Autodesk Fusion 360 part; units mm, degrees
note: some values were not read from the file. Set by a fixed rule: which sketch regions a step uses.
(part 11 of 59)
  spline S58 degree 5 poles (-18.7406, 34.6904) (-18.7407, 34.6905) (-18.7408, 34.6907) (-18.741, 34.6909) (-18.7414, 34.6913) (-18.7419, 34.6919) (-18.7424, 34.6925) (-18.7431, 34.6933) (-18.7438, 34.6941) (-18.7446, 34.695) (-18.7455, 34.696) (-18.7464, 34.697) (-18.7474, 34.6982) (-18.7485, 34.6994) (-18.7497, 34.7007) (-18.7509, 34.702) (-18.7522, 34.7035) (-18.7536, 34.705) (-18.755, 34.7066) (-18.7565, 34.7082) (-18.7581, 34.7099) (-18.7597, 34.7117) (-18.7615, 34.7136) (-18.7632, 34.7155) (-18.7651, 34.7175) (-18.767, 34.7195) (-18.769, 34.7216) (-18.771, 34.7238) (-18.7732, 34.726) (-18.7753, 34.7283) (-18.7776, 34.7307) (-18.7799, 34.7331) (-18.7823, 34.7355) (-18.7847, 34.738) (-18.7872, 34.7406) (-18.7897, 34.7433) (-18.7924, 34.7459) (-18.7951, 34.7487) (-18.7978, 34.7515) (-18.8006, 34.7543) (-18.8035, 34.7572) (-18.8064, 34.7602) (-18.8094, 34.7632) (-18.8124, 34.7662) (-18.8156, 34.7693) (-18.8187, 34.7725) (-18.822, 34.7757) (-18.8252, 34.7789) (-18.8286, 34.7822) (-18.832, 34.7855) (-18.8355, 34.7889) (-18.839, 34.7923) (-18.8426, 34.7958) (-18.8462, 34.7993) (-18.8499, 34.8029) (-18.8536, 34.8065) (-18.8574, 34.8101) (-18.8613, 34.8138) (-18.8652, 34.8175) (-18.8692, 34.8212) (-18.8732, 34.825) (-18.8773, 34.8289) (-18.8814, 34.8328) (-18.8856, 34.8367) (-18.8899, 34.8406) (-18.8942, 34.8446) (-18.8986, 34.8486) (-18.903, 34.8527) (-18.9074, 34.8568) (-18.9119, 34.8609) (-18.9165, 34.8651) (-18.9211, 34.8693) (-18.9258, 34.8736) (-18.9306, 34.8778) (-18.9353, 34.8821) (-18.9402, 34.8865) (-18.9451, 34.8909) (-18.95, 34.8953) (-18.955, 34.8997) (-18.96, 34.9042) (-18.9651, 34.9087) (-18.9703, 34.9132) (-18.9755, 34.9177) (-18.9807, 34.9223) (-18.986, 34.927) (-18.9914, 34.9316) (-18.9968, 34.9363) (-19.0022, 34.941) (-19.0077, 34.9457) (-19.0133, 34.9505) (-19.0189, 34.9553) (-19.0246, 34.9601) (-19.0303, 34.9649) (-19.036, 34.9698) (-19.0418, 34.9747) (-19.0477, 34.9796) (-19.0536, 34.9846) (-19.0595, 34.9895) (-19.0655, 34.9945) (-19.0715, 34.9996) (-19.0776, 35.0046) (-19.0838, 35.0097) (-19.09, 35.0148) (-19.0962, 35.0199) (-19.1025, 35.025) (-19.1088, 35.0302) (-19.1152, 35.0354) (-19.1216, 35.0406) (-19.1281, 35.0458) (-19.1346, 35.0511) (-19.1412, 35.0564) (-19.1478, 35.0617) (-19.1544, 35.067) (-19.1611, 35.0723) (-19.1679, 35.0777) (-19.1747, 35.083) (-19.1815, 35.0884) (-19.1884, 35.0939) (-19.1954, 35.0993) (-19.2024, 35.1048) (-19.2094, 35.1102) (-19.2165, 35.1157) (-19.2236, 35.1212) (-19.2307, 35.1268) (-19.2379, 35.1323) (-19.2452, 35.1379) (-19.2525, 35.1435) (-19.2598, 35.1491) (-19.2672, 35.1547) (-19.2747, 35.1603) (-19.2821, 35.166) (-19.2897, 35.1716) (-19.2972, 35.1773) (-19.3048, 35.183) (-19.3125, 35.1887) (-19.3202, 35.1945) (-19.3279, 35.2002) (-19.3357, 35.206) (-19.3436, 35.2118) (-19.3514, 35.2175) (-19.3593, 35.2233) (-19.3673, 35.2292) (-19.3753, 35.235) (-19.3834, 35.2408) (-19.3914, 35.2467) (-19.3996, 35.2526) (-19.4078, 35.2585) (-19.416, 35.2644) (-19.4242, 35.2703) (-19.4325, 35.2762) (-19.4409, 35.2822) (-19.4493, 35.2881) (-19.4577, 35.2941) (-19.4662, 35.3) (-19.4747, 35.306) (-19.4832, 35.312) (-19.4918, 35.318) (-19.5005, 35.3241) (-19.5091, 35.3301) (-19.5179, 35.3361) (-19.5266, 35.3422) (-19.5354, 35.3483) (-19.5443, 35.3543) (-19.5532, 35.3604) (-19.5621, 35.3665) (-19.5711, 35.3726) (-19.5801, 35.3787) (-19.5891, 35.3849) (-19.5982, 35.391) (-19.6073, 35.3971) (-19.6165, 35.4033) (-19.6257, 35.4095) (-19.635, 35.4156) (-19.6443, 35.4218) (-19.6536, 35.428) (-19.663, 35.4342) (-19.6724, 35.4404) (-19.6818, 35.4466) (-19.6913, 35.4528) (-19.7009, 35.4591) (-19.7104, 35.4653) (-19.72, 35.4715) (-19.7297, 35.4778) (-19.7394, 35.484) (-19.7491, 35.4903) (-19.7589, 35.4966) (-19.7687, 35.5029) (-19.7785, 35.5091) (-19.7884, 35.5154) (-19.7984, 35.5217) (-19.8083, 35.528) (-19.8183, 35.5343) (-19.8284, 35.5406) (-19.8384, 35.547) (-19.8486, 35.5533) (-19.8587, 35.5596) (-19.8689, 35.566) (-19.8791, 35.5723) (-19.8894, 35.5786) (-19.8997, 35.585) (-19.9101, 35.5914) (-19.9205, 35.5977) (-19.9309, 35.6041) (-19.9413, 35.6104) (-19.9518, 35.6168) (-19.9624, 35.6232) (-19.973, 35.6296) (-19.9836, 35.636) (-19.9942, 35.6423) (-20.0049, 35.6487) (-20.0156, 35.6551) (-20.0264, 35.6615) (-20.0372, 35.6679) (-20.048, 35.6743) (-20.0589, 35.6807) (-20.0698, 35.6872) (-20.0808, 35.6936) (-20.0917, 35.7) (-20.1028, 35.7064) (-20.1138, 35.7128) (-20.1249, 35.7193) (-20.136, 35.7257) (-20.1472, 35.7321) (-20.1584, 35.7385) (-20.1697, 35.745) (-20.1809, 35.7514) (-20.1922, 35.7578) (-20.2036, 35.7643) (-20.215, 35.7707) (-20.2264, 35.7771) (-20.2379, 35.7836) (-20.2493, 35.79) (-20.2609, 35.7965) (-20.2724, 35.8029) (-20.284, 35.8094) (-20.2957, 35.8158) (-20.3073, 35.8222) (-20.319, 35.8287) (-20.3308, 35.8351) (-20.3426, 35.8416) (-20.3544, 35.848) (-20.3639, 35.8532) (-20.371, 35.8571) (-20.3757, 35.8596) (-20.3781, 35.8609) knots 0 0 0 0 0 0 0.00416667 0.00833333 0.0125 0.01666667 0.02083333 0.025 0.02916667 0.03333333 0.0375 0.04166667 0.04583333 0.05 0.05416667 0.05833333 0.0625 0.06666667 0.07083333 0.075 0.07916667 0.08333333 0.0875 0.09166667 0.09583333 0.1 0.10416667 0.10833333 0.1125 0.11666667 0.12083333 0.125 0.12916667 0.13333333 0.1375 0.14166667 0.14583333 0.15 0.15416667 0.15833333 0.1625 0.16666667 0.17083333 0.175 0.17916667 0.18333333 0.1875 0.19166667 0.19583333 0.2 0.20416667 0.20833333 0.2125 0.21666667 0.22083333 0.225 0.22916667 0.23333333 0.2375 0.24166667 0.24583333 0.25 0.25416667 0.25833333 0.2625 0.26666667 0.27083333 0.275 0.27916667 0.28333333 0.2875 0.29166667 0.29583333 0.3 0.30416667 0.30833333 0.3125 0.31666667 0.32083333 0.325 0.32916667 0.33333333 0.3375 0.34166667 0.34583333 0.35 0.35416667 0.35833333 0.3625 0.36666667 0.37083333 0.375 0.37916667 0.38333333 0.3875 0.39166667 0.39583333 0.4 0.40416667 0.40833333 0.4125 0.41666667 0.42083333 0.425 0.42916667 0.43333333 0.4375 0.44166667 0.44583333 0.45 0.45416667 0.45833333 0.4625 0.46666667 0.47083333 0.475 0.47916667 0.48333333 0.4875 0.49166667 0.49583333 0.5 0.50416667 0.50833333 0.5125 0.51666667 0.52083333 0.525 0.52916667 0.53333333 0.5375 0.54166667 0.54583333 0.55 0.55416667 0.55833333 0.5625 0.56666667 0.57083333 0.575 0.57916667 0.58333333 0.5875 0.59166667 0.59583333 0.6 0.60416667 0.60833333 0.6125 0.61666667 0.62083333 0.625 0.62916667 0.63333333 0.6375 0.64166667 0.64583333 0.65 0.65416667 0.65833333 0.6625 0.66666667 0.67083333 0.675 0.67916667 0.68333333 0.6875 0.69166667 0.69583333 0.7 0.70416667 0.70833333 0.7125 0.71666667 0.72083333 0.725 0.72916667 0.73333333 0.7375 0.74166667 0.74583333 0.75 0.75416667 0.75833333 0.7625 0.76666667 0.77083333 0.775 0.77916667 0.78333333 0.7875 0.79166667 0.79583333 0.8 0.80416667 0.80833333 0.8125 0.81666667 0.82083333 0.825 0.82916667 0.83333333 0.8375 0.84166667 0.84583333 0.85 0.85416667 0.85833333 0.8625 0.86666667 0.87083333 0.875 0.87916667 0.88333333 0.8875 0.89166667 0.89583333 0.9 0.90416667 0.90833333 0.9125 0.91666667 0.92083333 0.925 0.92916667 0.93333333 0.9375 0.94166667 0.94583333 0.95 0.95416667 0.95833333 0.9625 0.96666667 0.97083333 0.975 0.97916667 0.98333333 0.9875 0.99166667 0.99583333 1 1 1 1 1 1
  line L121 (-6.937, 40.7047) -> (-6.9368, 40.7039)
  line L122 (-10.9659, 39.3948) -> (-10.9662, 39.3955)
  spline S59 degree 5 poles (-20.9575, 32.61) (-20.9576, 32.61) (-20.9577, 32.6102) (-20.958, 32.6104) (-20.9583, 32.6107) (-20.9589, 32.6112) (-20.9595, 32.6118) (-20.9602, 32.6125) (-20.961, 32.6132) (-20.9619, 32.614) (-20.9629, 32.6149) (-20.9639, 32.6159) (-20.9651, 32.6169) (-20.9663, 32.618) (-20.9675, 32.6192) (-20.9689, 32.6204) (-20.9704, 32.6217) (-20.9719, 32.623) (-20.9735, 32.6245) (-20.9752, 32.626) (-20.9769, 32.6275) (-20.9787, 32.6291) (-20.9806, 32.6308) (-20.9826, 32.6325) (-20.9847, 32.6343) (-20.9868, 32.6361) (-20.989, 32.638) (-20.9912, 32.6399) (-20.9936, 32.6419) (-20.996, 32.644) (-20.9984, 32.6461) (-21.001, 32.6482) (-21.0036, 32.6504) (-21.0063, 32.6527) (-21.009, 32.655) (-21.0119, 32.6573) (-21.0148, 32.6597) (-21.0177, 32.6622) (-21.0207, 32.6647) (-21.0238, 32.6672) (-21.027, 32.6698) (-21.0302, 32.6724) (-21.0335, 32.6751) (-21.0368, 32.6778) (-21.0403, 32.6806) (-21.0437, 32.6834) (-21.0473, 32.6862) (-21.0509, 32.6891) (-21.0546, 32.692) (-21.0583, 32.695) (-21.0621, 32.698) (-21.066, 32.701) (-21.0699, 32.7041) (-21.0739, 32.7072) (-21.0779, 32.7103) (-21.082, 32.7135) (-21.0862, 32.7167) (-21.0904, 32.72) (-21.0947, 32.7233) (-21.099, 32.7266) (-21.1034, 32.73) (-21.1079, 32.7333) (-21.1124, 32.7368) (-21.117, 32.7402) (-21.1216, 32.7437) (-21.1263, 32.7472) (-21.1311, 32.7508) (-21.1359, 32.7544) (-21.1408, 32.758) (-21.1457, 32.7616) (-21.1507, 32.7653) (-21.1557, 32.769) (-21.1608, 32.7727) (-21.166, 32.7765) (-21.1712, 32.7802) (-21.1764, 32.7841) (-21.1818, 32.7879) (-21.1871, 32.7918) (-21.1926, 32.7956) (-21.1981, 32.7996) (-21.2036, 32.8035) (-21.2092, 32.8075) (-21.2148, 32.8115) (-21.2205, 32.8155) (-21.2263, 32.8195) (-21.2321, 32.8236) (-21.238, 32.8277) (-21.2439, 32.8318) (-21.2498, 32.8359) (-21.2559, 32.8401) (-21.2619, 32.8442) (-21.2681, 32.8484) (-21.2742, 32.8527) (-21.2805, 32.8569) (-21.2867, 32.8612) (-21.2931, 32.8655) (-21.2995, 32.8698) (-21.3059, 32.8741) (-21.3124, 32.8784) (-21.3189, 32.8828) (-21.3255, 32.8872) (-21.3321, 32.8916) (-21.3388, 32.896) (-21.3455, 32.9004) (-21.3523, 32.9049) (-21.3592, 32.9094) (-21.3661, 32.9139) (-21.373, 32.9184) (-21.38, 32.9229) (-21.387, 32.9274) (-21.3941, 32.932) (-21.4012, 32.9366) (-21.4084, 32.9412) (-21.4156, 32.9458) (-21.4229, 32.9504) (-21.4302, 32.955) (-21.4376, 32.9597) (-21.445, 32.9644) (-21.4525, 32.969) (-21.46, 32.9737) (-21.4676, 32.9784) (-21.4752, 32.9832) (-21.4828, 32.9879) (-21.4905, 32.9927) (-21.4983, 32.9974) (-21.5061, 33.0022) (-21.5139, 33.007) (-21.5218, 33.0118) (-21.5297, 33.0166) (-21.5377, 33.0214) (-21.5458, 33.0263) (-21.5538, 33.0311) (-21.5619, 33.036) (-21.5701, 33.0409) (-21.5783, 33.0457) (-21.5866, 33.0506) (-21.5949, 33.0555) (-21.6032, 33.0605) (-21.6116, 33.0654) (-21.6201, 33.0703) (-21.6285, 33.0753) (-21.6371, 33.0802) (-21.6456, 33.0852) (-21.6542, 33.0902) (-21.6629, 33.0951) (-21.6716, 33.1001) (-21.6803, 33.1051) (-21.6891, 33.1101) (-21.698, 33.1152) (-21.7068, 33.1202) (-21.7158, 33.1252) (-21.7247, 33.1303) (-21.7337, 33.1353) (-21.7428, 33.1404) (-21.7519, 33.1454) (-21.761, 33.1505) (-21.7702, 33.1556) (-21.7794, 33.1607) (-21.7887, 33.1658) (-21.798, 33.1709) (-21.8073, 33.176) (-21.8167, 33.1811) (-21.8261, 33.1862) (-21.8356, 33.1913) (-21.8451, 33.1965) (-21.8547, 33.2016) (-21.8643, 33.2067) (-21.8739, 33.2119) (-21.8836, 33.217) (-21.8933, 33.2222) (-21.9031, 33.2274) (-21.9129, 33.2325) (-21.9228, 33.2377) (-21.9326, 33.2429) (-21.9426, 33.248) (-21.9525, 33.2532) (-21.9625, 33.2584) (-21.9726, 33.2636) (-21.9827, 33.2688) (-21.9928, 33.274) (-22.003, 33.2792) (-22.0132, 33.2844) (-22.0235, 33.2896) (-22.0337, 33.2948) (-22.0441, 33.3) (-22.0544, 33.3052) (-22.0649, 33.3105) (-22.0753, 33.3157) (-22.0858, 33.3209) (-22.0963, 33.3261) (-22.1069, 33.3313) (-22.1175, 33.3366) (-22.1281, 33.3418) (-22.1388, 33.347) (-22.1496, 33.3523) (-22.1603, 33.3575) (-22.1711, 33.3627) (-22.182, 33.368) (-22.1928, 33.3732) (-22.2038, 33.3784) (-22.2147, 33.3837) (-22.2257, 33.3889) (-22.2367, 33.3942) (-22.2478, 33.3994) (-22.2589, 33.4046) (-22.2701, 33.4099) (-22.2812, 33.4151) (-22.2925, 33.4204) (-22.3037, 33.4256) (-22.315, 33.4308) (-22.3264, 33.4361) (-22.3377, 33.4413) (-22.3491, 33.4466) (-22.3606, 33.4518) (-22.3721, 33.457) (-22.3836, 33.4623) (-22.3951, 33.4675) (-22.4067, 33.4727) (-22.4184, 33.478) (-22.43, 33.4832) (-22.4417, 33.4884) (-22.4535, 33.4937) (-22.4653, 33.4989) (-22.4771, 33.5041) (-22.4889, 33.5093) (-22.5008, 33.5145) (-22.5127, 33.5198) (-22.5247, 33.525) (-22.5367, 33.5302) (-22.5487, 33.5354) (-22.5608, 33.5406) (-22.5729, 33.5458) (-22.585, 33.551) (-22.5972, 33.5562) (-22.6094, 33.5614) (-22.6217, 33.5666) (-22.6339, 33.5718) (-22.6462, 33.577) (-22.6586, 33.5822) (-22.671, 33.5873) (-22.6834, 33.5925) (-22.6934, 33.5967) (-22.7009, 33.5998) (-22.7059, 33.6018) (-22.7084, 33.6029) knots 0 0 0 0 0 0 0.00416667 0.00833333 0.0125 0.01666667 0.02083333 0.025 0.02916667 0.03333333 0.0375 0.04166667 0.04583333 0.05 0.05416667 0.05833333 0.0625 0.06666667 0.07083333 0.075 0.07916667 0.08333333 0.0875 0.09166667 0.09583333 0.1 0.10416667 0.10833333 0.1125 0.11666667 0.12083333 0.125 0.12916667 0.13333333 0.1375 0.14166667 0.14583333 0.15 0.15416667 0.15833333 0.1625 0.16666667 0.17083333 0.175 0.17916667 0.18333333 0.1875 0.19166667 0.19583333 0.2 0.20416667 0.20833333 0.2125 0.21666667 0.22083333 0.225 0.22916667 0.23333333 0.2375 0.24166667 0.24583333 0.25 0.25416667 0.25833333 0.2625 0.26666667 0.27083333 0.275 0.27916667 0.28333333 0.2875 0.29166667 0.29583333 0.3 0.30416667 0.30833333 0.3125 0.31666667 0.32083333 0.325 0.32916667 0.33333333 0.3375 0.34166667 0.34583333 0.35 0.35416667 0.35833333 0.3625 0.36666667 0.37083333 0.375 0.37916667 0.38333333 0.3875 0.39166667 0.39583333 0.4 0.40416667 0.40833333 0.4125 0.41666667 0.42083333 0.425 0.42916667 0.43333333 0.4375 0.44166667 0.44583333 0.45 0.45416667 0.45833333 0.4625 0.46666667 0.47083333 0.475 0.47916667 0.48333333 0.4875 0.49166667 0.49583333 0.5 0.50416667 0.50833333 0.5125 0.51666667 0.52083333 0.525 0.52916667 0.53333333 0.5375 0.54166667 0.54583333 0.55 0.55416667 0.55833333 0.5625 0.56666667 0.57083333 0.575 0.57916667 0.58333333 0.5875 0.59166667 0.59583333 0.6 0.60416667 0.60833333 0.6125 0.61666667 0.62083333 0.625 0.62916667 0.63333333 0.6375 0.64166667 0.64583333 0.65 0.65416667 0.65833333 0.6625 0.66666667 0.67083333 0.675 0.67916667 0.68333333 0.6875 0.69166667 0.69583333 0.7 0.70416667 0.70833333 0.7125 0.71666667 0.72083333 0.725 0.72916667 0.73333333 0.7375 0.74166667 0.74583333 0.75 0.75416667 0.75833333 0.7625 0.76666667 0.77083333 0.775 0.77916667 0.78333333 0.7875 0.79166667 0.79583333 0.8 0.80416667 0.80833333 0.8125 0.81666667 0.82083333 0.825 0.82916667 0.83333333 0.8375 0.84166667 0.84583333 0.85 0.85416667 0.85833333 0.8625 0.86666667 0.87083333 0.875 0.87916667 0.88333333 0.8875 0.89166667 0.89583333 0.9 0.90416667 0.90833333 0.9125 0.91666667 0.92083333 0.925 0.92916667 0.93333333 0.9375 0.94166667 0.94583333 0.95 0.95416667 0.95833333 0.9625 0.96666667 0.97083333 0.975 0.97916667 0.98333333 0.9875 0.99166667 0.99583333 1 1 1 1 1 1
  line L123 (-9.8472, 39.8251) -> (-9.8469, 39.8243)
  arc A65 (-9.1146, 42.1298) -> (-10.0421, 41.8284) centre (0, 12.5) ccw
  line L124 (22.7115, -5.1281) -> (22.9441, -5.3086)
  arc A66 (21.9649, -6.0501) -> (22.7115, -5.1281) centre (0, 12.5) ccw
  line L125 (22.1898, -6.2401) -> (21.9649, -6.0501)
  line L126 (22.9441, -5.3086) -> (22.9448, -5.3091)
  line L127 (27.0473, 2.7529) -> (27.3243, 2.6531)
  spline S60 degree 5 poles (0.9213, 41.5307) (0.9213, 41.5307) (0.9213, 41.5309) (0.9213, 41.5313) (0.9213, 41.5318) (0.9213, 41.5325) (0.9213, 41.5334) (0.9214, 41.5344) (0.9214, 41.5355) (0.9214, 41.5367) (0.9214, 41.538) (0.9214, 41.5394) (0.9214, 41.5409) (0.9214, 41.5425) (0.9214, 41.5443) (0.9214, 41.5461) (0.9214, 41.5481) (0.9214, 41.5501) (0.9214, 41.5522) (0.9214, 41.5545) (0.9214, 41.5568) (0.9213, 41.5592) (0.9213, 41.5618) (0.9212, 41.5644) (0.9212, 41.5671) (0.9211, 41.5699) (0.9211, 41.5728) (0.921, 41.5758) (0.9209, 41.5788) (0.9208, 41.582) (0.9208, 41.5852) (0.9206, 41.5886) (0.9205, 41.592) (0.9204, 41.5955) (0.9203, 41.5991) (0.9201, 41.6028) (0.92, 41.6065) (0.9198, 41.6103) (0.9197, 41.6143) (0.9195, 41.6183) (0.9193, 41.6223) (0.9191, 41.6265) (0.9189, 41.6307) (0.9186, 41.635) (0.9184, 41.6394) (0.9182, 41.6439) (0.9179, 41.6484) (0.9176, 41.653) (0.9173, 41.6577) (0.917, 41.6624) (0.9167, 41.6673) (0.9164, 41.6722) (0.9161, 41.6771) (0.9157, 41.6822) (0.9153, 41.6873) (0.915, 41.6925) (0.9146, 41.6977) (0.9141, 41.703) (0.9137, 41.7084) (0.9133, 41.7139) (0.9128, 41.7194) (0.9124, 41.725) (0.9119, 41.7306) (0.9114, 41.7363) (0.9109, 41.7421) (0.9103, 41.748) (0.9098, 41.7539) (0.9092, 41.7599) (0.9087, 41.7659) (0.9081, 41.772) (0.9075, 41.7781) (0.9068, 41.7844) (0.9062, 41.7906) (0.9055, 41.797) (0.9049, 41.8034) (0.9042, 41.8099) (0.9035, 41.8164) (0.9027, 41.823) (0.902, 41.8296) (0.9012, 41.8363) (0.9005, 41.843) (0.8997, 41.8498) (0.8989, 41.8567) (0.898, 41.8636) (0.8972, 41.8706) (0.8963, 41.8777) (0.8954, 41.8847) (0.8945, 41.8919) (0.8936, 41.8991) (0.8927, 41.9063) (0.8917, 41.9137) (0.8907, 41.921) (0.8897, 41.9284) (0.8887, 41.9359) (0.8877, 41.9434) (0.8866, 41.951) (0.8856, 41.9586) (0.8845, 41.9663) (0.8834, 41.974) (0.8822, 41.9818) (0.8811, 41.9896) (0.8799, 41.9975) (0.8787, 42.0054) (0.8775, 42.0134) (0.8763, 42.0214) (0.875, 42.0295) (0.8738, 42.0376) (0.8725, 42.0458) (0.8712, 42.054) (0.8698, 42.0623) (0.8685, 42.0706) (0.8671, 42.0789) (0.8657, 42.0873) (0.8643, 42.0958) (0.8629, 42.1043) (0.8614, 42.1128) (0.86, 42.1214) (0.8585, 42.1301) (0.8569, 42.1388) (0.8554, 42.1475) (0.8538, 42.1563) (0.8523, 42.1651) (0.8507, 42.1739) (0.849, 42.1828) (0.8474, 42.1918) (0.8457, 42.2008) (0.844, 42.2098) (0.8423, 42.2189) (0.8406, 42.228) (0.8388, 42.2372) (0.8371, 42.2464) (0.8353, 42.2556) (0.8334, 42.2649) (0.8316, 42.2742) (0.8297, 42.2836) (0.8279, 42.293) (0.8259, 42.3025) (0.824, 42.312) (0.8221, 42.3215) (0.8201, 42.3311) (0.8181, 42.3407) (0.8161, 42.3503) (0.814, 42.36) (0.812, 42.3697) (0.8099, 42.3795) (0.8078, 42.3893) (0.8056, 42.3992) (0.8035, 42.409) (0.8013, 42.419) (0.7991, 42.4289) (0.7969, 42.4389) (0.7946, 42.449) (0.7923, 42.459) (0.79, 42.4691) (0.7877, 42.4793) (0.7854, 42.4895) (0.783, 42.4997) (0.7806, 42.5099) (0.7782, 42.5202) (0.7758, 42.5306) (0.7733, 42.5409) (0.7708, 42.5513) (0.7683, 42.5618) (0.7658, 42.5722) (0.7632, 42.5827) (0.7606, 42.5933) (0.758, 42.6038) (0.7554, 42.6145) (0.7528, 42.6251) (0.7501, 42.6358) (0.7474, 42.6465) (0.7447, 42.6572) (0.7419, 42.668) (0.7391, 42.6788) (0.7364, 42.6897) (0.7335, 42.7005) (0.7307, 42.7114) (0.7278, 42.7224) (0.7249, 42.7334) (0.722, 42.7444) (0.7191, 42.7554) (0.7161, 42.7665) (0.7131, 42.7776) (0.7101, 42.7887) (0.7071, 42.7999) (0.704, 42.8111) (0.7009, 42.8223) (0.6978, 42.8336) (0.6947, 42.8448) (0.6915, 42.8562) (0.6883, 42.8675) (0.6851, 42.8789) (0.6819, 42.8903) (0.6786, 42.9017) (0.6753, 42.9132) (0.672, 42.9247) (0.6687, 42.9362) (0.6653, 42.9478) (0.6619, 42.9594) (0.6585, 42.971) (0.6551, 42.9827) (0.6516, 42.9943) (0.6481, 43.006) (0.6446, 43.0178) (0.6411, 43.0295) (0.6375, 43.0413) (0.6339, 43.0531) (0.6303, 43.065) (0.6267, 43.0769) (0.623, 43.0888) (0.6193, 43.1007) (0.6156, 43.1126) (0.6118, 43.1246) (0.6081, 43.1366) (0.6043, 43.1487) (0.6005, 43.1607) (0.5966, 43.1728) (0.5927, 43.185) (0.5889, 43.1971) (0.5849, 43.2093) (0.581, 43.2215) (0.577, 43.2337) (0.573, 43.2459) (0.569, 43.2582) (0.5649, 43.2705) (0.5609, 43.2828) (0.5568, 43.2952) (0.5526, 43.3076) (0.5485, 43.32) (0.5443, 43.3324) (0.5401, 43.3448) (0.5359, 43.3573) (0.5316, 43.3698) (0.5273, 43.3823) (0.523, 43.3949) (0.5187, 43.4075) (0.5143, 43.4201) (0.5099, 43.4327) (0.5055, 43.4453) (0.5011, 43.458) (0.4966, 43.4707) (0.493, 43.4809) (0.4903, 43.4885) (0.4885, 43.4936) (0.4876, 43.4962) knots 0 0 0 0 0 0 0.00416667 0.00833333 0.0125 0.01666667 0.02083333 0.025 0.02916667 0.03333333 0.0375 0.04166667 0.04583333 0.05 0.05416667 0.05833333 0.0625 0.06666667 0.07083333 0.075 0.07916667 0.08333333 0.0875 0.09166667 0.09583333 0.1 0.10416667 0.10833333 0.1125 0.11666667 0.12083333 0.125 0.12916667 0.13333333 0.1375 0.14166667 0.14583333 0.15 0.15416667 0.15833333 0.1625 0.16666667 0.17083333 0.175 0.17916667 0.18333333 0.1875 0.19166667 0.19583333 0.2 0.20416667 0.20833333 0.2125 0.21666667 0.22083333 0.225 0.22916667 0.23333333 0.2375 0.24166667 0.24583333 0.25 0.25416667 0.25833333 0.2625 0.26666667 0.27083333 0.275 0.27916667 0.28333333 0.2875 0.29166667 0.29583333 0.3 0.30416667 0.30833333 0.3125 0.31666667 0.32083333 0.325 0.32916667 0.33333333 0.3375 0.34166667 0.34583333 0.35 0.35416667 0.35833333 0.3625 0.36666667 0.37083333 0.375 0.37916667 0.38333333 0.3875 0.39166667 0.39583333 0.4 0.40416667 0.40833333 0.4125 0.41666667 0.42083333 0.425 0.42916667 0.43333333 0.4375 0.44166667 0.44583333 0.45 0.45416667 0.45833333 0.4625 0.46666667 0.47083333 0.475 0.47916667 0.48333333 0.4875 0.49166667 0.49583333 0.5 0.50416667 0.50833333 0.5125 0.51666667 0.52083333 0.525 0.52916667 0.53333333 0.5375 0.54166667 0.54583333 0.55 0.55416667 0.55833333 0.5625 0.56666667 0.57083333 0.575 0.57916667 0.58333333 0.5875 0.59166667 0.59583333 0.6 0.60416667 0.60833333 0.6125 0.61666667 0.62083333 0.625 0.62916667 0.63333333 0.6375 0.64166667 0.64583333 0.65 0.65416667 0.65833333 0.6625 0.66666667 0.67083333 0.675 0.67916667 0.68333333 0.6875 0.69166667 0.69583333 0.7 0.70416667 0.70833333 0.7125 0.71666667 0.72083333 0.725 0.72916667 0.73333333 0.7375 0.74166667 0.74583333 0.75 0.75416667 0.75833333 0.7625 0.76666667 0.77083333 0.775 0.77916667 0.78333333 0.7875 0.79166667 0.79583333 0.8 0.80416667 0.80833333 0.8125 0.81666667 0.82083333 0.825 0.82916667 0.83333333 0.8375 0.84166667 0.84583333 0.85 0.85416667 0.85833333 0.8625 0.86666667 0.87083333 0.875 0.87916667 0.88333333 0.8875 0.89166667 0.89583333 0.9 0.90416667 0.90833333 0.9125 0.91666667 0.92083333 0.925 0.92916667 0.93333333 0.9375 0.94166667 0.94583333 0.95 0.95416667 0.95833333 0.9625 0.96666667 0.97083333 0.975 0.97916667 0.98333333 0.9875 0.99166667 0.99583333 1 1 1 1 1 1
  line L128 (-6.9368, -15.7039) -> (-6.937, -15.7047)
  spline S61 degree 5 poles (5.1346, -16.0878) (5.1347, -16.0879) (5.1347, -16.0881) (5.1348, -16.0884) (5.1349, -16.0889) (5.135, -16.0896) (5.1352, -16.0905) (5.1354, -16.0915) (5.1356, -16.0925) (5.1358, -16.0937) (5.1361, -16.095) (5.1363, -16.0964) (5.1367, -16.0979) (5.137, -16.0995) (5.1374, -16.1012) (5.1377, -16.103) (5.1381, -16.1049) (5.1386, -16.1069) (5.139, -16.1089) (5.1395, -16.1111) (5.14, -16.1134) (5.1406, -16.1158) (5.1411, -16.1182) (5.1417, -16.1208) (5.1423, -16.1234) (5.143, -16.1262) (5.1436, -16.129) (5.1443, -16.1319) (5.145, -16.1349) (5.1458, -16.1379) (5.1465, -16.1411) (5.1473, -16.1443) (5.1481, -16.1477) (5.149, -16.1511) (5.1499, -16.1545) (5.1508, -16.1581) (5.1517, -16.1617) (5.1527, -16.1655) (5.1536, -16.1693) (5.1546, -16.1731) (5.1557, -16.1771) (5.1567, -16.1811) (5.1578, -16.1852) (5.1589, -16.1893) (5.1601, -16.1936) (5.1613, -16.1979) (5.1625, -16.2023) (5.1637, -16.2067) (5.1649, -16.2112) (5.1662, -16.2158) (5.1675, -16.2205) (5.1689, -16.2252) (5.1702, -16.23) (5.1716, -16.2349) (5.173, -16.2398) (5.1745, -16.2448) (5.176, -16.2498) (5.1775, -16.2549) (5.179, -16.2601) (5.1806, -16.2654) (5.1822, -16.2707) (5.1838, -16.276) (5.1854, -16.2815) (5.1871, -16.2869) (5.1888, -16.2925) (5.1905, -16.2981) (5.1923, -16.3038) (5.1941, -16.3095) (5.1959, -16.3153) (5.1978, -16.3211) (5.1996, -16.327) (5.2015, -16.333) (5.2035, -16.339) (5.2054, -16.3451) (5.2074, -16.3512) (5.2094, -16.3573) (5.2115, -16.3636) (5.2136, -16.3699) (5.2157, -16.3762) (5.2178, -16.3826) (5.22, -16.389) (5.2222, -16.3955) (5.2244, -16.4021) (5.2266, -16.4087) (5.2289, -16.4153) (5.2312, -16.422) (5.2336, -16.4288) (5.2359, -16.4356) (5.2383, -16.4424) (5.2408, -16.4493) (5.2432, -16.4563) (5.2457, -16.4633) (5.2482, -16.4703) (5.2508, -16.4774) (5.2533, -16.4846) (5.2559, -16.4918) (5.2586, -16.499) (5.2612, -16.5063) (5.2639, -16.5136) (5.2666, -16.521) (5.2694, -16.5284) (5.2722, -16.5358) (5.275, -16.5433) (5.2778, -16.5509) (5.2807, -16.5585) (5.2836, -16.5661) (5.2865, -16.5738) (5.2895, -16.5815) (5.2925, -16.5893) (5.2955, -16.5971) (5.2986, -16.605) (5.3016, -16.6129) (5.3047, -16.6208) (5.3079, -16.6288) (5.3111, -16.6368) (5.3143, -16.6448) (5.3175, -16.6529) (5.3207, -16.6611) (5.324, -16.6692) (5.3273, -16.6775) (5.3307, -16.6857) (5.3341, -16.694) (5.3375, -16.7023) (5.3409, -16.7107) (5.3444, -16.7191) (5.3479, -16.7276) (5.3514, -16.7361) (5.355, -16.7446) (5.3586, -16.7531) (5.3622, -16.7617) (5.3658, -16.7704) (5.3695, -16.779) (5.3732, -16.7878) (5.377, -16.7965) (5.3807, -16.8053) (5.3846, -16.8141) (5.3884, -16.8229) (5.3922, -16.8318) (5.3961, -16.8407) (5.4001, -16.8497) (5.404, -16.8587) (5.408, -16.8677) (5.412, -16.8767) (5.4161, -16.8858) (5.4201, -16.895) (5.4242, -16.9041) (5.4284, -16.9133) (5.4325, -16.9225) (5.4367, -16.9318) (5.441, -16.941) (5.4452, -16.9504) (5.4495, -16.9597) (5.4538, -16.9691) (5.4582, -16.9785) (5.4625, -16.9879) (5.467, -16.9974) (5.4714, -17.0069) (5.4759, -17.0165) (5.4804, -17.026) (5.4849, -17.0356) (5.4895, -17.0452) (5.494, -17.0549) (5.4987, -17.0646) (5.5033, -17.0743) (5.508, -17.084) (5.5127, -17.0938) (5.5175, -17.1036) (5.5222, -17.1134) (5.527, -17.1233) (5.5319, -17.1332) (5.5367, -17.1431) (5.5416, -17.153) (5.5466, -17.163) (5.5515, -17.173) (5.5565, -17.183) (5.5615, -17.1931) (5.5666, -17.2032) (5.5717, -17.2133) (5.5768, -17.2234) (5.5819, -17.2336) (5.5871, -17.2437) (5.5923, -17.254) (5.5975, -17.2642) (5.6028, -17.2745) (5.6081, -17.2847) (5.6134, -17.2951) (5.6188, -17.3054) (5.6242, -17.3158) (5.6296, -17.3262) (5.635, -17.3366) (5.6405, -17.347) (5.646, -17.3575) (5.6515, -17.368) (5.6571, -17.3785) (5.6627, -17.389) (5.6683, -17.3996) (5.674, -17.4102) (5.6797, -17.4208) (5.6854, -17.4314) (5.6912, -17.4421) (5.697, -17.4527) (5.7028, -17.4634) (5.7086, -17.4742) (5.7145, -17.4849) (5.7204, -17.4957) (5.7263, -17.5065) (5.7323, -17.5173) (5.7383, -17.5281) (5.7443, -17.539) (5.7504, -17.5499) (5.7565, -17.5608) (5.7626, -17.5717) (5.7688, -17.5826) (5.7749, -17.5936) (5.7811, -17.6046) (5.7874, -17.6156) (5.7937, -17.6266) (5.8, -17.6377) (5.8063, -17.6487) (5.8127, -17.6598) (5.8191, -17.6709) (5.8255, -17.6821) (5.8319, -17.6932) (5.8384, -17.7044) (5.8449, -17.7156) (5.8515, -17.7268) (5.8581, -17.738) (5.8647, -17.7492) (5.8713, -17.7605) (5.878, -17.7718) (5.8847, -17.7831) (5.8914, -17.7944) (5.8982, -17.8058) (5.905, -17.8171) (5.9118, -17.8285) (5.9187, -17.8399) (5.9255, -17.8513) (5.9325, -17.8628) (5.9394, -17.8742) (5.9464, -17.8857) (5.9534, -17.8972) (5.959, -17.9064) (5.9633, -17.9133) (5.9661, -17.9179) (5.9675, -17.9202) knots 0 0 0 0 0 0 0.00416667 0.00833333 0.0125 0.01666667 0.02083333 0.025 0.02916667 0.03333333 0.0375 0.04166667 0.04583333 0.05 0.05416667 0.05833333 0.0625 0.06666667 0.07083333 0.075 0.07916667 0.08333333 0.0875 0.09166667 0.09583333 0.1 0.10416667 0.10833333 0.1125 0.11666667 0.12083333 0.125 0.12916667 0.13333333 0.1375 0.14166667 0.14583333 0.15 0.15416667 0.15833333 0.1625 0.16666667 0.17083333 0.175 0.17916667 0.18333333 0.1875 0.19166667 0.19583333 0.2 0.20416667 0.20833333 0.2125 0.21666667 0.22083333 0.225 0.22916667 0.23333333 0.2375 0.24166667 0.24583333 0.25 0.25416667 0.25833333 0.2625 0.26666667 0.27083333 0.275 0.27916667 0.28333333 0.2875 0.29166667 0.29583333 0.3 0.30416667 0.30833333 0.3125 0.31666667 0.32083333 0.325 0.32916667 0.33333333 0.3375 0.34166667 0.34583333 0.35 0.35416667 0.35833333 0.3625 0.36666667 0.37083333 0.375 0.37916667 0.38333333 0.3875 0.39166667 0.39583333 0.4 0.40416667 0.40833333 0.4125 0.41666667 0.42083333 0.425 0.42916667 0.43333333 0.4375 0.44166667 0.44583333 0.45 0.45416667 0.45833333 0.4625 0.46666667 0.47083333 0.475 0.47916667 0.48333333 0.4875 0.49166667 0.49583333 0.5 0.50416667 0.50833333 0.5125 0.51666667 0.52083333 0.525 0.52916667 0.53333333 0.5375 0.54166667 0.54583333 0.55 0.55416667 0.55833333 0.5625 0.56666667 0.57083333 0.575 0.57916667 0.58333333 0.5875 0.59166667 0.59583333 0.6 0.60416667 0.60833333 0.6125 0.61666667 0.62083333 0.625 0.62916667 0.63333333 0.6375 0.64166667 0.64583333 0.65 0.65416667 0.65833333 0.6625 0.66666667 0.67083333 0.675 0.67916667 0.68333333 0.6875 0.69166667 0.69583333 0.7 0.70416667 0.70833333 0.7125 0.71666667 0.72083333 0.725 0.72916667 0.73333333 0.7375 0.74166667 0.74583333 0.75 0.75416667 0.75833333 0.7625 0.76666667 0.77083333 0.775 0.77916667 0.78333333 0.7875 0.79166667 0.79583333 0.8 0.80416667 0.80833333 0.8125 0.81666667 0.82083333 0.825 0.82916667 0.83333333 0.8375 0.84166667 0.84583333 0.85 0.85416667 0.85833333 0.8625 0.86666667 0.87083333 0.875 0.87916667 0.88333333 0.8875 0.89166667 0.89583333 0.9 0.90416667 0.90833333 0.9125 0.91666667 0.92083333 0.925 0.92916667 0.93333333 0.9375 0.94166667 0.94583333 0.95 0.95416667 0.95833333 0.9625 0.96666667 0.97083333 0.975 0.97916667 0.98333333 0.9875 0.99166667 0.99583333 1 1 1 1 1 1
  arc A67 (-6.9214, -17.7174) -> (-5.9675, -17.9202) centre (0, 12.5) ccw
  spline S62 degree 5 poles (25.363, -5.3246) (25.3615, -5.3224) (25.3584, -5.3179) (25.3539, -5.3112) (25.3477, -5.3023) (25.3401, -5.2913) (25.3325, -5.2802) (25.3248, -5.2692) (25.3172, -5.2583) (25.3096, -5.2473) (25.3019, -5.2364) (25.2943, -5.2256) (25.2867, -5.2147) (25.2791, -5.2039) (25.2715, -5.1932) (25.2639, -5.1825) (25.2563, -5.1718) (25.2487, -5.1611) (25.2411, -5.1505) (25.2335, -5.1399) (25.2259, -5.1294) (25.2184, -5.1189) (25.2108, -5.1084) (25.2032, -5.098) (25.1957, -5.0876) (25.1881, -5.0772) (25.1806, -5.0669) (25.1731, -5.0566) (25.1655, -5.0464) (25.158, -5.0361) (25.1505, -5.026) (25.143, -5.0158) (25.1355, -5.0057) (25.128, -4.9956) (25.1205, -4.9856) (25.113, -4.9756) (25.1055, -4.9657) (25.0981, -4.9557) (25.0906, -4.9458) (25.0832, -4.936) (25.0757, -4.9262) (25.0683, -4.9164) (25.0609, -4.9067) (25.0534, -4.897) (25.046, -4.8873) (25.0386, -4.8777) (25.0312, -4.8681) (25.0238, -4.8585) (25.0165, -4.849) (25.0091, -4.8395) (25.0017, -4.8301) (24.9944, -4.8207) (24.9871, -4.8113) (24.9797, -4.802) (24.9724, -4.7927) (24.9651, -4.7835) (24.9578, -4.7743) (24.9505, -4.7651) (24.9432, -4.7559) (24.936, -4.7469) (24.9287, -4.7378) (24.9215, -4.7288) (24.9142, -4.7198) (24.907, -4.7108) (24.8998, -4.7019) (24.8926, -4.6931) (24.8854, -4.6842) (24.8782, -4.6754) (24.8711, -4.6667) (24.8639, -4.658) (24.8568, -4.6493) (24.8496, -4.6407) (24.8425, -4.6321) (24.8354, -4.6235) (24.8283, -4.615) (24.8212, -4.6065) (24.8142, -4.5981) (24.8071, -4.5897) (24.8001, -4.5813) (24.7931, -4.573) (24.7861, -4.5647) (24.7791, -4.5565) (24.7721, -4.5483) (24.7651, -4.5401) (24.7582, -4.532) (24.7512, -4.5239) (24.7443, -4.5159) (24.7374, -4.5079) (24.7305, -4.4999) (24.7236, -4.492) (24.7168, -4.4841) (24.7099, -4.4763) (24.7031, -4.4685) (24.6963, -4.4607) (24.6895, -4.453) (24.6827, -4.4453) (24.6759, -4.4377) (24.6692, -4.4301) (24.6625, -4.4225) (24.6558, -4.415) (24.6491, -4.4075) (24.6424, -4.4001) (24.6357, -4.3927) (24.6291, -4.3854) (24.6225, -4.3781) (24.6159, -4.3708) (24.6093, -4.3636) (24.6027, -4.3564) (24.5962, -4.3492) (24.5897, -4.3421) (24.5831, -4.3351) (24.5767, -4.3281) (24.5702, -4.3211) (24.5638, -4.3142) (24.5573, -4.3073) (24.5509, -4.3004) (24.5446, -4.2936) (24.5382, -4.2869) (24.5319, -4.2801) (24.5255, -4.2735) (24.5192, -4.2668) (24.513, -4.2602) (24.5067, -4.2537) (24.5005, -4.2472) (24.4943, -4.2407) (24.4881, -4.2343) (24.482, -4.2279) (24.4758, -4.2216) (24.4697, -4.2153) (24.4636, -4.2091) (24.4576, -4.2029) (24.4515, -4.1967) (24.4455, -4.1906) (24.4395, -4.1845) (24.4336, -4.1785) (24.4277, -4.1725) (24.4218, -4.1666) (24.4159, -4.1607) (24.41, -4.1549) (24.4042, -4.1491) (24.3984, -4.1433) (24.3926, -4.1376) (24.3869, -4.1319) (24.3812, -4.1263) (24.3755, -4.1207) (24.3698, -4.1152) (24.3642, -4.1097) (24.3586, -4.1043) (24.353, -4.0989) (24.3475, -4.0935) (24.342, -4.0882) (24.3365, -4.083) (24.3311, -4.0778) (24.3257, -4.0726) (24.3203, -4.0675) (24.3149, -4.0624) (24.3096, -4.0574) (24.3043, -4.0524) (24.2991, -4.0475) (24.2939, -4.0426) (24.2887, -4.0378) (24.2835, -4.033) (24.2784, -4.0282) (24.2733, -4.0236) (24.2683, -4.0189) (24.2633, -4.0143) (24.2583, -4.0098) (24.2534, -4.0053) (24.2485, -4.0008) (24.2436, -3.9964) (24.2388, -3.992) (24.234, -3.9877) (24.2293, -3.9835) (24.2246, -3.9793) (24.2199, -3.9751) (24.2153, -3.971) (24.2107, -3.9669) (24.2062, -3.9629) (24.2017, -3.959) (24.1972, -3.955) (24.1928, -3.9512) (24.1884, -3.9474) (24.1841, -3.9436) (24.1798, -3.9399) (24.1755, -3.9362) (24.1713, -3.9326) (24.1672, -3.9291) (24.1631, -3.9256) (24.159, -3.9221) (24.155, -3.9187) (24.151, -3.9153) (24.1471, -3.912) (24.1432, -3.9088) (24.1394, -3.9056) (24.1356, -3.9024) (24.1319, -3.8994) (24.1283, -3.8963) (24.1246, -3.8933) (24.1211, -3.8904) (24.1176, -3.8875) (24.1141, -3.8847) (24.1107, -3.8819) (24.1073, -3.8792) (24.104, -3.8766) (24.1008, -3.874) (24.0976, -3.8714) (24.0945, -3.8689) (24.0914, -3.8665) (24.0884, -3.8641) (24.0855, -3.8618) (24.0826, -3.8595) (24.0798, -3.8573) (24.077, -3.8551) (24.0743, -3.853) (24.0717, -3.851) (24.0691, -3.849) (24.0666, -3.8471) (24.0641, -3.8452) (24.0618, -3.8434) (24.0595, -3.8416) (24.0572, -3.8399) (24.0551, -3.8383) (24.053, -3.8367) (24.051, -3.8352) (24.049, -3.8338) (24.0471, -3.8324) (24.0453, -3.831) (24.0436, -3.8298) (24.042, -3.8286) (24.0404, -3.8274) (24.0389, -3.8263) (24.0375, -3.8253) (24.0362, -3.8244) (24.035, -3.8235) (24.0338, -3.8227) (24.0327, -3.8219) (24.0317, -3.8212) (24.0309, -3.8206) (24.0301, -3.82) (24.0294, -3.8195) (24.0287, -3.8191) (24.0283, -3.8188) (24.0281, -3.8186) (24.0279, -3.8185) (24.0278, -3.8184) knots -1 -1 -1 -1 -1 -1 -0.99583333 -0.99166667 -0.9875 -0.98333333 -0.97916667 -0.975 -0.97083333 -0.96666667 -0.9625 -0.95833333 -0.95416667 -0.95 -0.94583333 -0.94166667 -0.9375 -0.93333333 -0.92916667 -0.925 -0.92083333 -0.91666667 -0.9125 -0.90833333 -0.90416667 -0.9 -0.89583333 -0.89166667 -0.8875 -0.88333333 -0.87916667 -0.875 -0.87083333 -0.86666667 -0.8625 -0.85833333 -0.85416667 -0.85 -0.84583333 -0.84166667 -0.8375 -0.83333333 -0.82916667 -0.825 -0.82083333 -0.81666667 -0.8125 -0.80833333 -0.80416667 -0.8 -0.79583333 -0.79166667 -0.7875 -0.78333333 -0.77916667 -0.775 -0.77083333 -0.76666667 -0.7625 -0.75833333 -0.75416667 -0.75 -0.74583333 -0.74166667 -0.7375 -0.73333333 -0.72916667 -0.725 -0.72083333 -0.71666667 -0.7125 -0.70833333 -0.70416667 -0.7 -0.69583333 -0.69166667 -0.6875 -0.68333333 -0.67916667 -0.675 -0.67083333 -0.66666667 -0.6625 -0.65833333 -0.65416667 -0.65 -0.64583333 -0.64166667 -0.6375 -0.63333333 -0.62916667 -0.625 -0.62083333 -0.61666667 -0.6125 -0.60833333 -0.60416667 -0.6 -0.59583333 -0.59166667 -0.5875 -0.58333333 -0.57916667 -0.575 -0.57083333 -0.56666667 -0.5625 -0.55833333 -0.55416667 -0.55 -0.54583333 -0.54166667 -0.5375 -0.53333333 -0.52916667 -0.525 -0.52083333 -0.51666667 -0.5125 -0.50833333 -0.50416667 -0.5 -0.49583333 -0.49166667 -0.4875 -0.48333333 -0.47916667 -0.475 -0.47083333 -0.46666667 -0.4625 -0.45833333 -0.45416667 -0.45 -0.44583333 -0.44166667 -0.4375 -0.43333333 -0.42916667 -0.425 -0.42083333 -0.41666667 -0.4125 -0.40833333 -0.40416667 -0.4 -0.39583333 -0.39166667 -0.3875 -0.38333333 -0.37916667 -0.375 -0.37083333 -0.36666667 -0.3625 -0.35833333 -0.35416667 -0.35 -0.34583333 -0.34166667 -0.3375 -0.33333333 -0.32916667 -0.325 -0.32083333 -0.31666667 -0.3125 -0.30833333 -0.30416667 -0.3 -0.29583333 -0.29166667 -0.2875 -0.28333333 -0.27916667 -0.275 -0.27083333 -0.26666667 -0.2625 -0.25833333 -0.25416667 -0.25 -0.24583333 -0.24166667 -0.2375 -0.23333333 -0.22916667 -0.225 -0.22083333 -0.21666667 -0.2125 -0.20833333 -0.20416667 -0.2 -0.19583333 -0.19166667 -0.1875 -0.18333333 -0.17916667 -0.175 -0.17083333 -0.16666667 -0.1625 -0.15833333 -0.15416667 -0.15 -0.14583333 -0.14166667 -0.1375 -0.13333333 -0.12916667 -0.125 -0.12083333 -0.11666667 -0.1125 -0.10833333 -0.10416667 -0.1 -0.09583333 -0.09166667 -0.0875 -0.08333333 -0.07916667 -0.075 -0.07083333 -0.06666667 -0.0625 -0.05833333 -0.05416667 -0.05 -0.04583333 -0.04166667 -0.0375 -0.03333333 -0.02916667 -0.025 -0.02083333 -0.01666667 -0.0125 -0.00833333 -0.00416667 0 0 0 0 0 0
  line L129 (12.6491, -13.6453) -> (12.5209, -13.3803)
  line L130 (26.1453, -0.1491) -> (26.1461, -0.1495)
  line L131 (3.9507, -16.2745) -> (3.9106, -15.9828)
  arc A68 (2.755, -18.3773) -> (3.7249, -18.2754) centre (0, 12.5) ccw
  spline S63 degree 5 poles (22.9448, -5.3091) (22.9448, -5.3092) (22.945, -5.3093) (22.9453, -5.3095) (22.9457, -5.3098) (22.9463, -5.3103) (22.9469, -5.3108) (22.9477, -5.3114) (22.9486, -5.312) (22.9496, -5.3127) (22.9506, -5.3135) (22.9518, -5.3144) (22.953, -5.3153) (22.9543, -5.3162) (22.9557, -5.3172) (22.9572, -5.3183) (22.9588, -5.3195) (22.9604, -5.3207) (22.9622, -5.3219) (22.964, -5.3232) (22.9659, -5.3246) (22.9679, -5.326) (22.9699, -5.3274) (22.9721, -5.3289) (22.9743, -5.3305) (22.9766, -5.3321) (22.979, -5.3337) (22.9814, -5.3354) (22.984, -5.3372) (22.9866, -5.3389) (22.9893, -5.3408) (22.992, -5.3427) (22.9948, -5.3446) (22.9978, -5.3465) (23.0007, -5.3485) (23.0038, -5.3506) (23.0069, -5.3527) (23.0101, -5.3548) (23.0134, -5.357) (23.0167, -5.3592) (23.0201, -5.3614) (23.0236, -5.3637) (23.0271, -5.366) (23.0308, -5.3683) (23.0344, -5.3707) (23.0382, -5.3731) (23.042, -5.3756) (23.0459, -5.3781) (23.0499, -5.3806) (23.0539, -5.3831) (23.058, -5.3857) (23.0621, -5.3883) (23.0664, -5.391) (23.0706, -5.3937) (23.075, -5.3964) (23.0794, -5.3991) (23.0839, -5.4019) (23.0884, -5.4047) (23.093, -5.4075) (23.0977, -5.4103) (23.1024, -5.4132) (23.1072, -5.4161) (23.1121, -5.4191) (23.117, -5.422) (23.122, -5.425) (23.127, -5.428) (23.1321, -5.431) (23.1373, -5.4341) (23.1425, -5.4372) (23.1478, -5.4403) (23.1531, -5.4434) (23.1585, -5.4466) (23.164, -5.4497) (23.1695, -5.4529) (23.1751, -5.4562) (23.1807, -5.4594) (23.1864, -5.4627) (23.1921, -5.4659) (23.1979, -5.4692) (23.2038, -5.4726) (23.2097, -5.4759) (23.2157, -5.4793) (23.2217, -5.4826) (23.2278, -5.486) (23.234, -5.4895) (23.2402, -5.4929) (23.2464, -5.4963) (23.2527, -5.4998) (23.2591, -5.5033) (23.2655, -5.5068) (23.272, -5.5103) (23.2785, -5.5139) (23.2851, -5.5174) (23.2918, -5.521) (23.2984, -5.5246) (23.3052, -5.5282) (23.312, -5.5318) (23.3188, -5.5354) (23.3257, -5.539) (23.3327, -5.5427) (23.3397, -5.5464) (23.3468, -5.5501) (23.3539, -5.5538) (23.361, -5.5575) (23.3683, -5.5612) (23.3755, -5.5649) (23.3828, -5.5687) (23.3902, -5.5724) (23.3976, -5.5762) (23.4051, -5.58) (23.4126, -5.5838) (23.4202, -5.5876) (23.4278, -5.5914) (23.4355, -5.5952) (23.4432, -5.5991) (23.451, -5.6029) (23.4588, -5.6068) (23.4666, -5.6106) (23.4746, -5.6145) (23.4825, -5.6184) (23.4905, -5.6223) (23.4986, -5.6262) (23.5067, -5.6301) (23.5149, -5.634) (23.5231, -5.6379) (23.5313, -5.6419) (23.5396, -5.6458) (23.548, -5.6498) (23.5564, -5.6537) (23.5648, -5.6577) (23.5733, -5.6617) (23.5818, -5.6657) (23.5904, -5.6696) (23.5991, -5.6736) (23.6077, -5.6776) (23.6165, -5.6816) (23.6252, -5.6857) (23.634, -5.6897) (23.6429, -5.6937) (23.6518, -5.6977) (23.6607, -5.7018) (23.6697, -5.7058) (23.6788, -5.7098) (23.6879, -5.7139) (23.697, -5.7179) (23.7062, -5.722) (23.7154, -5.726) (23.7247, -5.7301) (23.734, -5.7342) (23.7433, -5.7383) (23.7527, -5.7423) (23.7622, -5.7464) (23.7716, -5.7505) (23.7812, -5.7546) (23.7907, -5.7587) (23.8004, -5.7627) (23.81, -5.7668) (23.8197, -5.7709) (23.8295, -5.775) (23.8393, -5.7791) (23.8491, -5.7832) (23.859, -5.7873) (23.8689, -5.7914) (23.8788, -5.7955) (23.8888, -5.7996) (23.8989, -5.8038) (23.909, -5.8079) (23.9191, -5.812) (23.9292, -5.8161) (23.9395, -5.8202) (23.9497, -5.8243) (23.96, -5.8284) (23.9703, -5.8325) (23.9807, -5.8366) (23.9911, -5.8408) (24.0016, -5.8449) (24.0121, -5.849) (24.0226, -5.8531) (24.0332, -5.8572) (24.0438, -5.8613) (24.0545, -5.8654) (24.0652, -5.8695) (24.0759, -5.8736) (24.0867, -5.8777) (24.0975, -5.8818) (24.1084, -5.8859) (24.1193, -5.89) (24.1302, -5.8941) (24.1412, -5.8982) (24.1522, -5.9023) (24.1633, -5.9064) (24.1744, -5.9105) (24.1855, -5.9146) (24.1967, -5.9187) (24.2079, -5.9228) (24.2191, -5.9269) (24.2304, -5.9309) (24.2417, -5.935) (24.2531, -5.9391) (24.2645, -5.9431) (24.276, -5.9472) (24.2874, -5.9513) (24.299, -5.9553) (24.3105, -5.9594) (24.3221, -5.9634) (24.3337, -5.9675) (24.3454, -5.9715) (24.3571, -5.9756) (24.3689, -5.9796) (24.3806, -5.9836) (24.3925, -5.9877) (24.4043, -5.9917) (24.4162, -5.9957) (24.4281, -5.9997) (24.4401, -6.0037) (24.4521, -6.0077) (24.4642, -6.0117) (24.4762, -6.0157) (24.4884, -6.0197) (24.5005, -6.0237) (24.5127, -6.0277) (24.5249, -6.0316) (24.5372, -6.0356) (24.5495, -6.0395) (24.5618, -6.0435) (24.5742, -6.0475) (24.5866, -6.0514) (24.599, -6.0553) (24.6115, -6.0593) (24.624, -6.0632) (24.6365, -6.0671) (24.6491, -6.071) (24.6617, -6.0749) (24.6744, -6.0788) (24.6871, -6.0827) (24.6998, -6.0866) (24.7125, -6.0905) (24.7253, -6.0943) (24.7382, -6.0982) (24.751, -6.1021) (24.7639, -6.1059) (24.7743, -6.109) (24.782, -6.1113) (24.7872, -6.1128) (24.7898, -6.1136) knots 0 0 0 0 0 0 0.00416667 0.00833333 0.0125 0.01666667 0.02083333 0.025 0.02916667 0.03333333 0.0375 0.04166667 0.04583333 0.05 0.05416667 0.05833333 0.0625 0.06666667 0.07083333 0.075 0.07916667 0.08333333 0.0875 0.09166667 0.09583333 0.1 0.10416667 0.10833333 0.1125 0.11666667 0.12083333 0.125 0.12916667 0.13333333 0.1375 0.14166667 0.14583333 0.15 0.15416667 0.15833333 0.1625 0.16666667 0.17083333 0.175 0.17916667 0.18333333 0.1875 0.19166667 0.19583333 0.2 0.20416667 0.20833333 0.2125 0.21666667 0.22083333 0.225 0.22916667 0.23333333 0.2375 0.24166667 0.24583333 0.25 0.25416667 0.25833333 0.2625 0.26666667 0.27083333 0.275 0.27916667 0.28333333 0.2875 0.29166667 0.29583333 0.3 0.30416667 0.30833333 0.3125 0.31666667 0.32083333 0.325 0.32916667 0.33333333 0.3375 0.34166667 0.34583333 0.35 0.35416667 0.35833333 0.3625 0.36666667 0.37083333 0.375 0.37916667 0.38333333 0.3875 0.39166667 0.39583333 0.4 0.40416667 0.40833333 0.4125 0.41666667 0.42083333 0.425 0.42916667 0.43333333 0.4375 0.44166667 0.44583333 0.45 0.45416667 0.45833333 0.4625 0.46666667 0.47083333 0.475 0.47916667 0.48333333 0.4875 0.49166667 0.49583333 0.5 0.50416667 0.50833333 0.5125 0.51666667 0.52083333 0.525 0.52916667 0.53333333 0.5375 0.54166667 0.54583333 0.55 0.55416667 0.55833333 0.5625 0.56666667 0.57083333 0.575 0.57916667 0.58333333 0.5875 0.59166667 0.59583333 0.6 0.60416667 0.60833333 0.6125 0.61666667 0.62083333 0.625 0.62916667 0.63333333 0.6375 0.64166667 0.64583333 0.65 0.65416667 0.65833333 0.6625 0.66666667 0.67083333 0.675 0.67916667 0.68333333 0.6875 0.69166667 0.69583333 0.7 0.70416667 0.70833333 0.7125 0.71666667 0.72083333 0.725 0.72916667 0.73333333 0.7375 0.74166667 0.74583333 0.75 0.75416667 0.75833333 0.7625 0.76666667 0.77083333 0.775 0.77916667 0.78333333 0.7875 0.79166667 0.79583333 0.8 0.80416667 0.80833333 0.8125 0.81666667 0.82083333 0.825 0.82916667 0.83333333 0.8375 0.84166667 0.84583333 0.85 0.85416667 0.85833333 0.8625 0.86666667 0.87083333 0.875 0.87916667 0.88333333 0.8875 0.89166667 0.89583333 0.9 0.90416667 0.90833333 0.9125 0.91666667 0.92083333 0.925 0.92916667 0.93333333 0.9375 0.94166667 0.94583333 0.95 0.95416667 0.95833333 0.9625 0.96666667 0.97083333 0.975 0.97916667 0.98333333 0.9875 0.99166667 0.99583333 1 1 1 1 1 1
  line L132 (13.578, -12.8417) -> (13.7171, -13.1012)
  line L133 (-5.1345, -16.087) -> (-5.0824, -15.7972)
  line L134 (28.2039, 19.4368) -> (27.918, 19.3665)
  arc A69 (-8.0125, -15.1109) -> (-6.8665, -15.418) centre (0, 12.5) ccw
  arc A70 (0.9119, -16.2355) -> (2.0967, -16.1734) centre (0, 12.5) ccw
  line L135 (5.1345, -16.087) -> (5.1346, -16.0878)
  line L136 (26.8948, 1.5341) -> (26.6221, 1.6453)
  arc A71 (3.9106, -15.9828) -> (5.0824, -15.7972) centre (0, 12.5) ccw
  line L137 (5.0824, -15.7972) -> (5.1345, -16.087)
  line L138 (28.2047, 19.437) -> (28.2039, 19.4368)
  line L139 (-5.1346, -16.0878) -> (-5.1345, -16.087)